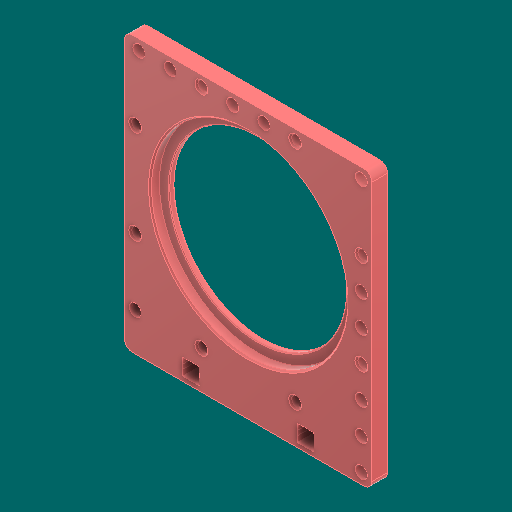
# Autodesk Inventor part: Baseplate
Saved by Autodesk Inventor 2023.1 (Build 271208000, 208)
## iProperties
Created: 2022-10-30
Part Number: Baseplate
Material: ABS Plastic
Document SubType Name: Modeling
Designer: zac-h
Density: 1.06 g/cm^3
Appearance: Smooth - Red
Author: zac-h
## iProperties of the stored document Baseplate_3DPrint.ipt
Created: 2022-10-31
Part Number: Baseplate_3DPrint
Material: Generic
Document SubType Name: Modeling
Designer: zac-h
Density: 1 g/cm^3
Appearance: Default
Author: zac-h
Autodesk Inventor part; units mm, degrees
ref_plane "YZ Plane" through (0, 0, 0) normal (1, 0, 0) x (0, 1, 0)
ref_plane "XZ Plane" through (0, 0, 0) normal (0, 1, 0) x (-1, 0, 0)
ref_plane "XY Plane" through (0, 0, 0) normal (0, 0, 1) x (1, 0, 0)
sketch "Sketch1" plane through (0, 0, 0) normal (0, 1, 0) x (-1, 0, 0)
  line L0 (36, 0) -> (42.827628, 0) construction
  line L1 (39.925, 2.54) -> (39.925, 6.35)
  line L2 (39.925, 6.35) -> (41.08, 6.35)
  line L3 (0, 0) -> (0, -85.525839) construction
  line L4 (39.925, 2.54) -> (0, 2.54) construction
  line L5 (0, 0) -> (36, 0) construction
  line L6 (41.08, 6.35) -> (41.08, 0)
  line L7 (41.08, 0) -> (36, 0)
  line L8 (39.925, 2.54) -> (36, 2.54)
  line L9 (36, 2.54) -> (36, 0)
  dimension "d2" = 79.85
  dimension "d5" = 6.35
  dimension "d7" = 5.08
  dimension "d74" = 2.54
  dimension "d79" = 72
  constraints: 20 end point, 4 horizontal, 4 vertical, 2 perpendicular, 1 point on line
  measures "d2" diameter of L1.start L3
  measures "d5" distance between parallel lines of L2 L0
  measures "d7" horizontal distance of L2.end L0.start
  measures "d74" distance between parallel lines of L0 L8
  measures "d79" diameter of L9 L3
revolve "Revolution1" add sketch "Sketch1" angle 360 about axis through (0, 0, 0) along (0, 0, -1)
sketch "Sketch2" plane through (0, 0, 0) normal (0, 0, -1) x (-1, 0, 0)
  circle A0 centre (45.990768, 19.05) radius 1.984375
  circle A1 centre (45.990768, 19.05) radius 4.314
  circle A2 centre (0, 0) radius 49.780049 construction
  circle A3 centre (0, 0) radius 38.1 construction
  circle A4 centre (-23.328382, -56.319696) radius 15.24 construction
  circle A5 centre (23.328382, -56.319696) radius 15.24 construction
  line L0 (-26.630382, -53.017696) -> (-20.026382, -53.017696)
  line L1 (-20.026382, -53.017696) -> (-20.026382, -59.621696)
  line L2 (-20.026382, -59.621696) -> (-26.630382, -59.621696)
  line L3 (-26.630382, -59.621696) -> (-26.630382, -53.017696)
  line L4 (-26.630382, -53.017696) -> (-20.026382, -59.621696) construction
  line L5 (-20.026382, -53.017696) -> (-26.630382, -59.621696) construction
  line L6 (20.026382, -53.017696) -> (26.630382, -53.017696)
  line L7 (26.630382, -53.017696) -> (26.630382, -59.621696)
  line L8 (26.630382, -59.621696) -> (20.026382, -59.621696)
  line L9 (20.026382, -59.621696) -> (20.026382, -53.017696)
  line L10 (20.026382, -53.017696) -> (26.630382, -59.621696) construction
  line L11 (26.630382, -53.017696) -> (20.026382, -59.621696) construction
  circle A6 centre (0, 0) radius 45.72 construction
  line L12 (0, 0) -> (45.990768, 19.05) construction
  line L13 (0, 0) -> (69.635584, 0) construction
  circle A7 centre (19.05, 45.990768) radius 1.984375
  circle A8 centre (19.05, 45.990768) radius 4.314
  circle A9 centre (-19.05, 45.990768) radius 1.984375
  circle A10 centre (-19.05, 45.990768) radius 4.314
  circle A11 centre (-45.990768, 19.05) radius 1.984375
  circle A12 centre (-45.990768, 19.05) radius 4.314
  circle A13 centre (-45.990768, -19.05) radius 1.984375
  circle A14 centre (-45.990768, -19.05) radius 4.314
  circle A15 centre (-19.05, -45.990768) radius 1.984375
  circle A16 centre (-19.05, -45.990768) radius 4.314
  circle A17 centre (19.05, -45.990768) radius 1.984375
  circle A18 centre (19.05, -45.990768) radius 4.314
  circle A19 centre (45.990768, -19.05) radius 1.984375
  circle A20 centre (45.990768, -19.05) radius 4.314
  line L14 (-40.328382, -72.619696) -> (-6.328382, -72.619696) construction
  line L15 (-6.328382, -72.619696) -> (-6.328382, -14.619696) construction
  line L16 (-6.328382, -14.619696) -> (-40.328382, -14.619696) construction
  line L17 (-40.328382, -14.619696) -> (-40.328382, -72.619696) construction
  line L18 (-40.328382, -72.619696) -> (-6.328382, -14.619696) construction
  line L19 (-6.328382, -72.619696) -> (-40.328382, -14.619696) construction
  circle A21 centre (-23.328382, -43.619696) radius 12.7 construction
  circle A22 centre (-23.328382, -56.319696) radius 3.429
  line L20 (-50.304768, 50.304768) -> (50.304768, 50.304768)
  line L21 (50.304768, 50.304768) -> (50.304768, -61.464)
  line L22 (50.304768, -61.464) -> (-50.304768, -61.464)
  line L23 (-50.304768, -61.464) -> (-50.304768, 50.304768)
  line L24 (-19.05, 45.990768) -> (-45.990768, 45.990768) construction
  line L25 (-45.990768, 45.990768) -> (-45.990768, 19.05) construction
  circle A23 centre (-45.990768, 45.990768) radius 2.413
  circle A24 centre (-45.990768, 45.990768) radius 4.314
  line L26 (-45.990768, -19.05) -> (-45.990768, -31.75) construction
  circle A25 centre (-45.990768, -31.75) radius 2.413
  circle A26 centre (-45.990768, -44.45) radius 2.413
  circle A27 centre (-45.990768, -57.15) radius 2.413
  line L27 (-45.990768, 19.05) -> (-45.990768, -19.05) construction
  line L28 (-19.05, 45.990768) -> (-6.35, 45.990768) construction
  circle A28 centre (-6.35, 45.990768) radius 2.413
  line L29 (19.05, 45.990768) -> (6.35, 45.990768) construction
  circle A29 centre (6.35, 45.990768) radius 2.413
  line L30 (19.05, 45.990768) -> (31.75, 45.990768) construction
  circle A30 centre (31.75, 45.990768) radius 2.413
  circle A31 centre (44.45, 45.990768) radius 2.413
  circle A32 centre (-45.990768, -57.15) radius 4.314
  circle A33 centre (23.328382, -56.319696) radius 5.144304
  circle A34 centre (44.45, 45.990768) radius 4.314
  line L31 (48.756962, 46.237088) -> (50.29773, 19.296319)
  circle A35 centre (0, 0) radius 40.799078
  circle A36 centre (-45.990768, -6.35) radius 2.413
  circle A37 centre (-45.990768, 6.35) radius 2.413
  circle A38 centre (23.328382, -56.319696) radius 3.429
  circle A39 centre (45.990768, -45.990768) radius 2.413
  circle A40 centre (45.990768, -45.990768) radius 4.191 construction
  line L32 (-23.328382, -56.319696) -> (0, 0) construction
  line L33 (23.328382, -56.319696) -> (0, 0) construction
  point P0 (27.555707, -59.251177)
  point P1 (49.718811, -21.220783)
  point P2 (-20.026382, -55.395122)
  point P3 (-20.026382, -57.24427)
  point P4 (-22.403808, -59.621696)
  point P5 (-24.252956, -59.621696)
  point P6 (-26.630382, -57.24427)
  point P7 (-26.630382, -55.395122)
  point P8 (-24.252956, -53.017696)
  point P9 (-22.403808, -53.017696)
  point P10 (23.328382, -61.464)
  point P11 (50.304768, -19.05)
  point P12 (50.304768, 19.05)
  point P13 (44.45, 50.304768)
  point P14 (-45.990768, 50.304768)
  point P15 (-50.304768, 45.990768)
  point P16 (-50.304768, -57.15)
  point P17 (-45.990768, -61.464)
  point P18 (24.252956, -59.621696)
  point P19 (22.403808, -59.621696)
  point P20 (20.026382, -57.24427)
  point P21 (20.026382, -55.395122)
  point P22 (22.403808, -53.017696)
  point P23 (24.252956, -53.017696)
  point P24 (26.630382, -57.24427)
  point P25 (26.630382, -55.395122)
  dimension "d10" = 8.628
  dimension "d31" = 25.4
  dimension "d9" = 3.96875
  dimension "d16" = 76.2
  dimension "d17" = 30.48
  dimension "d18" = 6.604
  dimension "d19" = 6.604
  dimension "d20" = 6.604
  dimension "d21" = 6.604
  dimension "d24" = 22.5
  dimension "d27" = 360
  dimension "d29" = 34
  dimension "d30" = 58
  dimension "d32" = 6.858
  dimension "d35" = 38.1
  dimension "d36" = 4.826
  dimension "d37" = 12.7
  dimension "d38" = 4.826
  dimension "d41" = 12.7
  dimension "d48" = 12.7
  dimension "d49" = 4.826
  dimension "d50" = 12.7
  dimension "d51" = 12.7
  dimension "d54" = 12.7
  dimension "d66" = 90
  dimension "d71" = 4.826
  dimension "d72" = 91.44
  dimension "d73" = 8.382
  constraints: 68 end point, 35 centre point, 23 coincident, 12 horizontal, 8 parallel, 7 tangent, 6 midpoint, 5 perpendicular, 4 equal radius, 3 vertical, 3 vertical alignment, 2 horizontal alignment, 1 point on line, 63 other
  measures "d9" diameter of A0
  measures "d16" diameter of A3
  measures "d17" diameter of A4
  measures "d18" distance of L1.end L2.end
  measures "d19" distance of L0.end L1.end
  measures "d20" distance of L7.end L8.end
  measures "d21" distance of L6.end L7.end
  measures "d24" angle of L13 L12
  measures "d29" distance of L16.end L15.end
  measures "d30" distance of L16.end L14.start
  measures "d32" diameter of A22
  measures "d35" distance of A7.centre L24.start
  measures "d36" diameter of A23
  measures "d37" distance of L26.start L26.end
  measures "d38" diameter of A25
  measures "d41" distance of A25.centre A26.centre
  measures "d48" distance of L24.start L28.end
  measures "d49" diameter of A28
  measures "d50" distance of L29.start L29.end
  measures "d51" distance of L29.start L30.end
  measures "d54" distance of A30.centre A31.centre
  measures "d71" diameter of A39
  measures "d72" diameter of A6
  measures "d73" diameter of A40
extrude "Extrusion1" add sketch "Sketch2" against normal blind 6.35 contours A1 | A8 | A10 | A12 | A14 | A33 | A20 | L21 L22 A32 L23 A24 L20 A34 L31 A1 | A1 L31 A34 L20 L21 | A34 | L22 L23 A32 | A32 | A24 L23 L20 | A24 | A16 | A18
chamfer "Chamfer1" distance 0.6 angle 45 1 edges at (36, 0, 0)
chamfer "Chamfer2" distance 0.6 angle 45 15 edges at (-44.0064, 19.05, 6.35) (-44.0064, -19.05, 6.35) (-17.0656, -45.9908, 6.35) (21.0344, -45.9908, 6.35) (47.9751, -19.05, 6.35) (47.9751, 19.05, 6.35) (21.0344, 45.9908, 6.35) (-17.0656, 45.9908, 6.35) (-17.0656, 45.9908, 0) (-44.0064, 19.05, 0) (-44.0064, -19.05, 0) (-17.0656, -45.9908, 0) (21.0344, -45.9908, 0) (47.9751, -19.05, 0) (47.9751, 19.05, 0)
chamfer "Chamfer3" distance 0.3 angle 45 1 edges at (36, 0, 2.54)
chamfer "Chamfer4" distance 0.6 angle 45 1 edges at (39.925, 0, 6.35)
fillet "Fillet1" radius 3.175 4 edges at (-50.3048, -61.464, 3.175) (-50.3048, 50.3048, 3.175) (50.3048, 50.3048, 3.175) (50.3048, -61.464, 3.175)
body "Solid1"
